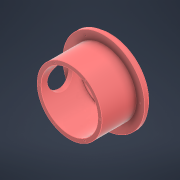
# Autodesk Inventor part: 021
Saved by Autodesk Inventor 2022 (Build 260153000, 153)
## iProperties
Created: 2021-11-06
Part Number: 021
Material: Stainless Steel, 440C
Document SubType Name: Modeling
Designer: vinicius.miguel
Density: 7.75 g/cm^3
Appearance: Smooth - Red
Mass: 1109.64 g
Surface Area: 482.868 cm^2
Volume: 143.18 cm^3
Author: vinicius.miguel
Autodesk Inventor part; units mm, degrees
ref_plane "XZ Plane" through (0, 0, 0) normal (0, 1, 0) x (-1, 0, 0)
ref_plane "XY Plane" through (0, 0, 0) normal (0, 0, 1) x (1, 0, 0)
sketch "Sketch1" plane through (0, 0, 0) normal (1, 0, 0) x (0, 1, 0)
  line L0 (0, 0) -> (0, 16.4674) construction
  line L1 (-57, -4.6) -> (-57, 0)
  line L2 (-57, 0) -> (-60, 0)
  line L3 (-60, 0) -> (-60, 5.4)
  line L4 (-60, 5.4) -> (-44.45, 5.4)
  line L5 (-44.45, 5.4) -> (-44.45, 2)
  line L6 (-44.45, 2) -> (-41, 2)
  line L7 (-41, 2) -> (-41, 1)
  line L8 (-41, 1) -> (-39, 1)
  line L9 (-39, 1) -> (-39, 2)
  line L10 (-39, 2) -> (-37, 2)
  line L11 (-37, -4.6) -> (-57, -4.6)
  line L12 (-37, -4.6) -> (-37, 2)
  line L13 (-47.5, 5.4) -> (-47.5, 55.4)
  line L14 (-47.5, 55.4) -> (-41.5, 55.4)
  line L15 (-41.5, 55.4) -> (-41.5, 2)
  point P0 (-47.5615, 5.4)
  dimension "d2" = 4.6
  dimension "d3" = 10
  dimension "d4" = 1
  dimension "d5" = 2
  dimension "d8" = 88.9
  dimension "d9" = 120
  dimension "d19" = 74
  dimension "d20" = 114
  dimension "d21" = 2
  dimension "d22" = 78
  dimension "d40" = 2
  dimension "d44" = 83
  dimension "d45" = 60
  dimension "d46" = 6
  constraints: 32 end point, 10 perpendicular, 4 point on line, 3 vertical, 1 horizontal alignment
  measures "d2" distance of L1.start L1.end
  measures "d3" distance between parallel lines of L4 L11
  measures "d4" distance of L8.end L9.end
  measures "d5" distance of L7.end L8.end
  measures "d8" diameter of L5 L0
  measures "d9" diameter of L3 L0
  measures "d19" diameter of L12 L0
  measures "d20" diameter of L1 L0
  measures "d21" distance of L9.end L10.end
  measures "d22" diameter of L9 L0
  measures "d40" distance between parallel lines of L2 L6
  measures "d44" diameter of L15 L0
  measures "d45" distance between parallel lines of L11 L14
  measures "d46" distance of L13.end L14.end
revolve "Revolution1" add sketch "Sketch1" angle 360 about axis through (0, 0, 0) along (0, 0, 1)
chamfer "Chamfer4" distance 1 angle 45 1 edges at (0, 57, -4.6)
sketch "Sketch2" plane through (0, 0, -4.6) normal (0, 0, -1) x (-1, 0, 0)
  point P0 (0, 0)
  point P1 (-53, 0)
  dimension "d26" = 53
  constraints: 1 horizontal alignment
  measures "d26" distance of point (0, 0) point (-53, 0)
hole "Hole1" at (53, 0, -4.6) direction (0, 0, 1) diameter 2.459 end through all counterbore diameter 4 counterbore depth 4.6 thread size "M3x0.5" class "6H" standard "ANSI Metric M Profile"
pattern_circular "Circular Pattern1" count 3 over 360 about axis through (0, 0, 2.7) along (0, 0, 1) of "Hole1"
chamfer "Chamfer5" distance 3 angle 45 1 edges at (0, 37, -4.6)
sketch "Sketch3" plane through (0, 0, 55.4) normal (0, 0, 1) x (1, 0, 0)
  circle A0 centre (0, 0) radius 47.5 projected
  circle A1 centre (0, 0) radius 41.5 projected
  circle A2 centre (0, 0) radius 47.5 projected
  point P0 (44.5, 0)
  dimension "d65" = 44.5
  constraints: 1 horizontal alignment
  measures "d65" distance of point (44.5, 0) point (0, 0)
hole "Hole2" at (44.5, 0, 55.4) direction (0, 0, -1) diameter 2.459 depth 8.8 tip angle 118 thread size "M3x0.5" class "6H" standard "ISO Metric profile"
pattern_circular "Circular Pattern2" count 6 over 360 about axis through (0, 0, 30.4) along (0, 0, 1) of "Hole2"
ref_plane "Work Plane1" through (-47.5, 0, 30.4) normal (1, 0, 0) x (0, 1, 0)
sketch "Sketch4" plane through (-47.5, 0, 30.4) normal (1, 0, 0) x (0, 1, 0)
  circle A0 centre (0, -3) radius 19
  line L0 (60, -25) -> (-60, -25) projected
  point P0 (0, -30.4)
  dimension "d57" = 38
  dimension "d58" = 22
  constraints: 1 centre point, 1 vertical alignment
  measures "d57" diameter of A0
  measures "d58" distance from line of A0.centre L0
extrude "Extrusion1" cut sketch "Sketch4" along normal blind 15
chamfer "Chamfer6" distance 0.25 angle 45 4 edges at (0, 47.5, 55.4) (0, 41.5, 55.4) (0, 60, 5.4) (0, 60, 0)
body "Solid1"
